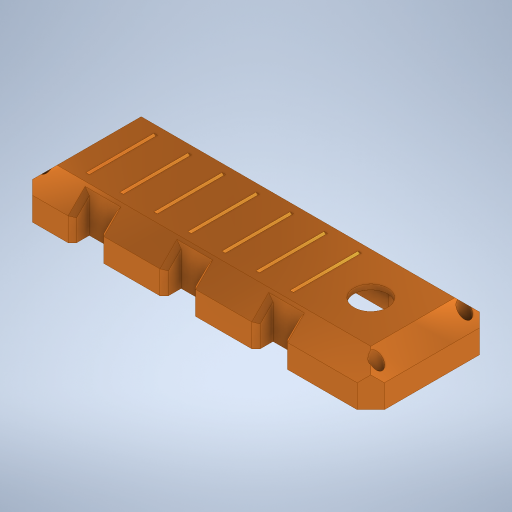
# Autodesk Inventor part: TapaSujecion
Saved by Autodesk Inventor 2024.2 (Build 282272000, 272)
## iProperties
Created: 2024-08-12
Part Number: TapaSujecion
Material: Generic
Document SubType Name: Modeling
Designer: Admin
Density: 1 g/cm^3
Appearance: Metal 1600F Hot
Author: Admin
Autodesk Inventor part; units mm, degrees
ref_plane "YZ Plane" through (0, 0, 0) normal (1, 0, 0) x (0, 1, 0)
ref_plane "XZ Plane" through (0, 0, 0) normal (0, 1, 0) x (-1, 0, 0)
ref_plane "XY Plane" through (0, 0, 0) normal (0, 0, 1) x (1, 0, 0)
sketch "Sketch1" plane through (0, 0, 0) normal (0, 1, 0) x (-1, 0, 0)
  line L0 (-95.5, 36) -> (95.5, 36)
  line L1 (103.5, 28) -> (103.5, -28)
  line L2 (95.5, -36) -> (-95.5, -36)
  line L3 (-103.5, -28) -> (-103.5, 28)
  line L4 (-103.5, 36) -> (103.5, -36) construction
  line L5 (103.5, 36) -> (-103.5, -36) construction
  line L6 (95.5, 36) -> (103.5, 28)
  line L7 (103.5, -28) -> (95.5, -36)
  line L8 (-103.5, -28) -> (-95.5, -36)
  line L9 (-95.5, 36) -> (-103.5, 28)
  point P0 (0, 0)
  dimension "d0" = 72
  dimension "d1" = 207
  dimension "d2" = 8
  dimension "d3" = 8
  dimension "d4" = 8
  dimension "d5" = 8
  dimension "d6" = 8
  dimension "d7" = 8
  dimension "d8" = 8
  dimension "d9" = 8
  constraints: 20 end point, 8 point on line, 2 midpoint, 2 parallel, 1 horizontal, 1 perpendicular
  measures "d0" distance of L5.start L4.end
  measures "d1" distance of L4.end L5.end
  measures "d2" distance of L0.end L5.start
  measures "d3" distance of L1.start L5.start
  measures "d4" distance of L1.end L4.end
  measures "d5" distance of L2.start L4.end
  measures "d6" distance of L3.start L5.end
  measures "d7" distance of L2.end L5.end
  measures "d8" distance of L0.start L4.start
  measures "d9" distance of L3.end L4.start
extrude "Extrusion1" add sketch "Sketch1" along normal blind 25
chamfer "Chamfer2" distance 11.3 angle 45 4 edges at (0, 25, 36) (-103.5, 25, 0) (0, 25, -36) (103.5, 25, 0)
shell "Shell1" thickness 3 removed faces 1 at (-31.8333, 0, -12)
sketch "Sketch3" plane through (0, 25, 0) normal (0, 1, 0) x (1, 0, 0)
  line L0 (103.5, -28) -> (103.5, 28) projected
  line L1 (103.5, 0) -> (67.5, 0)
  circle A0 centre (67.5, 0) radius 9.925
  point P0 (0, 0)
  dimension "d23" = 36
  dimension "d24" = 19.85
  constraints: 2 end point, 1 centre point, 1 coincident, 1 horizontal, 1 midpoint
  measures "d23" distance of L1.start L1.end
  measures "d24" diameter of A0
extrude "EspacioSwitch" cut sketch "Sketch3" against normal blind 3
sketch "Sketch4" plane through (0, 0, 0) normal (0, -1, 0) x (1, 0, 0)
  line L0 (-97.3787, -29.8787) -> (-97.3787, 29.8787) construction
  circle A0 centre (-97.3787, -25.8787) radius 1.7
  circle A1 centre (-97.3787, -25.8787) radius 5
  line L1 (-103.5, 0) -> (-108.5, 0) construction
  circle A2 centre (-97.3787, 25.8787) radius 1.7
  circle A3 centre (-97.3787, 25.8787) radius 5
  line L2 (-103.5, 28) -> (-95.5, 36) projected
  line L3 (-95.5, 36) -> (-60.5, 36) construction
  line L4 (-95.5, 36) -> (95.5, 36) projected
  circle A4 centre (96.6213, 25.8787) radius 5
  circle A5 centre (96.6213, 25.8787) radius 1.7
  circle A6 centre (96.6213, -25.8787) radius 5
  circle A7 centre (96.6213, -25.8787) radius 1.7
  point P0 (0, 0)
  point P1 (-97.3787, -29.8787)
  dimension "d27" = 10
  dimension "d28" = 3.4
  dimension "d29" = 4
  dimension "d39" = 194
  constraints: 8 centre point, 6 end point, 4 coincident, 2 horizontal, 2 point on line, 2 symmetric about line, 1 vertical, 10 other
  measures "d27" diameter of A1
  measures "d28" diameter of A0
  measures "d29" distance of point (-97.379, -29.879) A0.centre
  measures "d39" distance of A3.centre A4.centre
extrude "Extrusion4" add sketch "Sketch4" against normal through all
extrude "Extrusion5" cut sketch "Sketch4" against normal through all contours A0 | A2 | A5 | A7
sketch "Sketch5" plane through (0, 25, 0) normal (0, 1, 0) x (1, 0, 0)
  circle A0 centre (-97.3787, 25.8787) radius 1.7 projected
  circle A1 centre (-97.3787, 25.8787) radius 3.5
  line L0 (-103.5, 28) -> (-103.5, -28) projected
  line L1 (-103.5, 0) -> (-92.2, 0) construction
  line L2 (-92.2, -24.7) -> (-92.2, 24.7) projected
  circle A2 centre (-97.3787, -25.8787) radius 3.5
  line L3 (0, 0) -> (0, -20) construction
  circle A3 centre (96.6213, -25.8787) radius 3.5
  circle A4 centre (96.6213, 25.8787) radius 3.5
  line L4 (90.5, 0) -> (101.8, 0) construction
  dimension "d35" = 7
  dimension "d47" = 194
  constraints: 6 end point, 4 centre point, 2 midpoint, 1 coincident, 1 collinear, 1 horizontal, 1 symmetric about line, 1 vertical, 7 other
  measures "d35" diameter of A1
  measures "d47" distance of A2.centre A3.centre
extrude "Extrusion6" cut sketch "Sketch5" against normal blind 12
sketch "Sketch7" plane through (0, 0, 0) normal (0, -1, 0) x (1, 0, 0)
  line L0 (95.5, -36) -> (-95.5, -36) projected
  line L1 (-72, -36) -> (-56, -36)
  line L2 (-56, -36) -> (-56, -26)
  line L3 (-56, -26) -> (-72, -26)
  line L4 (-72, -26) -> (-72, -36)
  line L5 (-103.5, -28) -> (-103.5, 28) projected
  line L6 (0, 0) -> (-10, 0) construction
  line L7 (-18, -36) -> (-2, -36)
  line L8 (-2, -36) -> (-2, -26)
  line L9 (-2, -26) -> (-18, -26)
  line L10 (-18, -26) -> (-18, -36)
  line L11 (36, -36) -> (52, -36)
  line L12 (52, -36) -> (52, -26)
  line L13 (52, -26) -> (36, -26)
  line L14 (36, -26) -> (36, -36)
  line L15 (-72, 36) -> (-56, 36)
  line L16 (-56, 36) -> (-56, 26)
  line L17 (-56, 26) -> (-72, 26)
  line L18 (-72, 26) -> (-72, 36)
  line L19 (-18, 36) -> (-2, 36)
  line L20 (-2, 36) -> (-2, 26)
  line L21 (-2, 26) -> (-18, 26)
  line L22 (-18, 26) -> (-18, 36)
  line L23 (36, 36) -> (52, 36)
  line L24 (52, 36) -> (52, 26)
  line L25 (52, 26) -> (36, 26)
  line L26 (36, 26) -> (36, 36)
  line L27 (-75, -23) -> (-53, -23)
  line L28 (-53, -23) -> (-53, -39)
  line L29 (-53, -39) -> (-75, -39)
  line L30 (-75, -39) -> (-75, -23)
  line L31 (1, -23) -> (1, -39)
  line L32 (1, -39) -> (-21, -39)
  line L33 (-21, -23) -> (1, -23)
  line L34 (-21, -39) -> (-21, -23)
  line L35 (55, -23) -> (55, -39)
  line L36 (55, -39) -> (33, -39)
  line L37 (33, -23) -> (55, -23)
  line L38 (33, -39) -> (33, -23)
  line L39 (-75, 23) -> (-53, 23)
  line L40 (-53, 23) -> (-53, 39)
  line L41 (-53, 39) -> (-75, 39)
  line L42 (-75, 39) -> (-75, 23)
  line L43 (1, 23) -> (1, 39)
  line L44 (1, 39) -> (-21, 39)
  line L45 (-21, 23) -> (1, 23)
  line L46 (-21, 39) -> (-21, 23)
  line L47 (55, 23) -> (55, 39)
  line L48 (55, 39) -> (33, 39)
  line L49 (33, 23) -> (55, 23)
  line L50 (33, 39) -> (33, 23)
  line L51 (-95.5, 36) -> (95.5, 36) projected
  line L52 (55, 36) -> (-75, 36)
  line L53 (-75, -36) -> (55, -36)
  point P0 (33, 36)
  point P1 (-53, -36)
  point P2 (-75, 36)
  point P3 (-53, 36)
  point P4 (-21, 36)
  point P5 (1, 36)
  point P6 (1, -36)
  point P7 (-21, -36)
  point P8 (33, -36)
  dimension "d54" = 16
  dimension "d55" = 10
  dimension "d57" = 31.5
  dimension "d61" = 54
  dimension "d66" = 3
  dimension "d69" = 54
  constraints: 102 end point, 24 symmetric about line, 7 point on line, 4 horizontal, 4 parallel, 3 perpendicular, 37 other
  measures "d54" distance of L2.end L3.end
  measures "d55" distance of L3.end L1.start
  measures "d57" distance between parallel lines of L5 L4
  measures "d61" distance of L1.start L7.start
  measures "d66" distance between parallel lines of L3 L27
  measures "d69" distance of L27.end L31.start
extrude "Extrusion7" cut sketch "Sketch7" against normal blind 30 contours L0 L14 L13 L12 | L0 L10 L9 L8 | L0 L4 L3 L2 | L15 L16 L17 L18 | L19 L20 L21 L22 | L23 L24 L25 L26
extrude "Extrusion8" add sketch "Sketch7" against normal through all contours L0 L12 L13 L14 L38 L37 L35 | L8 L9 L10 L0 L34 L33 L31 | L2 L3 L4 L0 L30 L27 L28 | L18 L17 L16 L51 L40 L39 L42 | L22 L21 L20 L51 L43 L45 L46 | L26 L25 L24 L51 L47 L49 L50
chamfer "Chamfer3" distance 2.5 angle 45 24 edges at (-72, 18.7, 31) (-56, 18.7, 31) (-56, 6.85, 36) (-72, 6.85, 36) (-56, 18.7, -31) (-72, 18.7, -31) (-72, 6.85, -36) (-56, 6.85, -36) (-18, 18.7, -31) (-2, 18.7, -31) (-2, 6.85, -36) (-18, 6.85, -36) (36, 6.85, -36) (36, 18.7, -31) (52, 18.7, -31) (52, 6.85, -36) (-18, 18.7, 31) (-2, 18.7, 31) (-18, 6.85, 36) (-2, 6.85, 36) (36, 6.85, 36) (36, 18.7, 31) (52, 18.7, 31) (52, 6.85, 36)
sketch "Sketch10" plane through (0, 0, 0) normal (0, 0, 1) x (1, 0, 0)
  line L0 (92.2, 25) -> (-92.2, 25) projected
  line L1 (0, 25) -> (2, 25)
  line L2 (2, 25) -> (5.5753, 22)
  line L3 (2, 25) -> (6.6672, 25) construction
  line L4 (5.5753, 22) -> (3.5753, 22)
  line L5 (3.5753, 22) -> (0, 25)
  line L6 (-20, 25) -> (-18, 25)
  line L7 (-16.4247, 22) -> (-20, 25)
  line L8 (-18, 25) -> (-14.4247, 22)
  line L9 (-14.4247, 22) -> (-16.4247, 22)
  line L10 (-40, 25) -> (-38, 25)
  line L11 (-36.4247, 22) -> (-40, 25)
  line L12 (-38, 25) -> (-34.4247, 22)
  line L13 (-34.4247, 22) -> (-36.4247, 22)
  line L14 (-60, 25) -> (-58, 25)
  line L15 (-56.4247, 22) -> (-60, 25)
  line L16 (-58, 25) -> (-54.4247, 22)
  line L17 (-54.4247, 22) -> (-56.4247, 22)
  line L18 (-80, 25) -> (-78, 25)
  line L19 (-76.4247, 22) -> (-80, 25)
  line L20 (-78, 25) -> (-74.4247, 22)
  line L21 (-74.4247, 22) -> (-76.4247, 22)
  line L22 (20, 25) -> (22, 25)
  line L23 (23.5753, 22) -> (20, 25)
  line L24 (22, 25) -> (25.5753, 22)
  line L25 (25.5753, 22) -> (23.5753, 22)
  line L26 (0, 25) -> (2, 25)
  line L27 (3.5753, 22) -> (0, 25)
  line L28 (2, 25) -> (5.5753, 22)
  line L29 (5.5753, 22) -> (3.5753, 22)
  line L30 (-20, 25) -> (-18, 25)
  line L31 (-16.4247, 22) -> (-20, 25)
  line L32 (-18, 25) -> (-14.4247, 22)
  line L33 (-14.4247, 22) -> (-16.4247, 22)
  line L34 (-40, 25) -> (-38, 25)
  line L35 (-36.4247, 22) -> (-40, 25)
  line L36 (-38, 25) -> (-34.4247, 22)
  line L37 (-34.4247, 22) -> (-36.4247, 22)
  line L38 (-60, 25) -> (-58, 25)
  line L39 (-56.4247, 22) -> (-60, 25)
  line L40 (-58, 25) -> (-54.4247, 22)
  line L41 (-54.4247, 22) -> (-56.4247, 22)
  line L42 (40, 25) -> (42, 25)
  line L43 (43.5753, 22) -> (40, 25)
  line L44 (42, 25) -> (45.5753, 22)
  line L45 (45.5753, 22) -> (43.5753, 22)
  line L46 (20, 25) -> (22, 25)
  line L47 (23.5753, 22) -> (20, 25)
  line L48 (22, 25) -> (25.5753, 22)
  line L49 (25.5753, 22) -> (23.5753, 22)
  line L50 (0, 25) -> (2, 25)
  line L51 (3.5753, 22) -> (0, 25)
  line L52 (2, 25) -> (5.5753, 22)
  line L53 (5.5753, 22) -> (3.5753, 22)
  line L54 (-20, 25) -> (-18, 25)
  line L55 (-16.4247, 22) -> (-20, 25)
  line L56 (-18, 25) -> (-14.4247, 22)
  line L57 (-14.4247, 22) -> (-16.4247, 22)
  line L58 (-40, 25) -> (-38, 25)
  line L59 (-36.4247, 22) -> (-40, 25)
  line L60 (-38, 25) -> (-34.4247, 22)
  line L61 (-34.4247, 22) -> (-36.4247, 22)
  point P0 (0, 0)
  dimension "d83" = 2
  dimension "d85" = 40
  dimension "d86" = 2
  dimension "d87" = 3
  dimension "d90" = 20
  dimension "d93" = 20
  constraints: 122 end point, 4 horizontal, 1 equal length, 1 midpoint, 1 point on line, 112 other
  measures "d83" distance of L1.start L1.end
  measures "d85" angle of L2 L3
  measures "d86" distance of L2.end L4.end
  measures "d87" distance between parallel lines of L4 L0
  measures "d90" distance of L1.start L6.start
  measures "d93" distance of L1.start L22.start
extrude "Extrusion9" cut sketch "Sketch10" along normal mid plane 40
equation "\"d3\" = d2"
equation "\"d4\" = d2"
equation "\"d5\" = d4"
equation "\"d7\" = d6"
equation "\"d9\" = d8"
body "Solid1"
